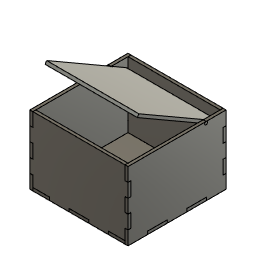
ex7 (Autodesk Fusion 360 design; units mm, degrees)
Autodesk Fusion 360 part; units mm, degrees
sketch "Sketch1" plane through (0, 0, 0) normal (1, 0, 0) x (0, 0, -1) in component "Component"
  line L0 (0, 0) -> (-100, 0)
  line L1 (-100, 0) -> (-100, 70)
  line L2 (-100, 70) -> (0, 70)
  line L3 (0, 70) -> (0, 0)
  line L4 (0, 3) -> (-100, 3)
  line L5 (-3, -14) -> (-3, 70)
  line L6 (-97, 70) -> (-97, 0)
  line L7 (-20, 3) -> (-40, 3)
  line L8 (-40, 3) -> (-40, 0)
  line L9 (-40, 0) -> (-20, 0)
  line L10 (-20, 0) -> (-20, 3)
  line L11 (-60, 3) -> (-80, 3)
  line L12 (-80, 3) -> (-80, 0)
  line L13 (-80, 0) -> (-60, 0)
  line L14 (-60, 0) -> (-60, 3)
  line L15 (-97, 14) -> (-100, 14)
  line L16 (-100, 14) -> (-100, 28)
  line L17 (-100, 28) -> (-97, 28)
  line L18 (-97, 28) -> (-97, 14)
  line L19 (-100, 42) -> (-97, 42)
  line L20 (-97, 42) -> (-97, 56)
  line L21 (-97, 56) -> (-100, 56)
  line L22 (-100, 56) -> (-100, 42)
  line L23 (0, 56) -> (-3, 56)
  line L24 (-3, 56) -> (-3, 42)
  line L25 (-3, 42) -> (0, 42)
  line L26 (0, 42) -> (0, 56)
  line L27 (-3, 28) -> (0, 28)
  line L28 (0, 28) -> (0, 14)
  line L29 (0, 14) -> (-3, 14)
  line L30 (-3, 14) -> (-3, 28)
  circle A0 centre (-20.404, 68.5087) radius 1.5
  dimension "d5" = 100
  dimension "d6" = 70
  dimension "d9" = 3
  dimension "d10" = 3
  dimension "d11" = 3
  dimension "d12" = 14
  dimension "d13" = 14
  dimension "d14" = 14
  dimension "d15" = 14
  dimension "d16" = 14
  dimension "d17" = 14
  dimension "d18" = 14
  dimension "d19" = 14
  dimension "d20" = 20
  dimension "d21" = 20
  dimension "d22" = 20
  dimension "d23" = 20
  dimension "d67" = 3
  constraint horizontal L0
  constraint vertical L1
  constraint horizontal L2
  constraint vertical L3
  constraint coincident L0.start L3.end
  constraint coincident L1 L4.end
  constraint perpendicular L1 L4
  constraint coincident L2 L5.end
  constraint perpendicular L2 L5
  constraint coincident L2 L6.start
  constraint coincident L0 L6.end
  constraint perpendicular L0 L6
  constraint horizontal L7
  constraint vertical L8
  constraint horizontal L9
  constraint vertical L10
  constraint coincident L0 L8.end
  constraint coincident L4 L7.start
  constraint horizontal L11
  constraint vertical L12
  constraint horizontal L13
  constraint vertical L14
  constraint coincident L0 L12.end
  constraint coincident L4 L11.start
  constraint horizontal L15
  constraint vertical L16
  constraint horizontal L17
  constraint vertical L18
  constraint coincident L1 L16.end
  constraint coincident L6 L15.start
  constraint horizontal L19
  constraint vertical L20
  constraint horizontal L21
  constraint vertical L22
  constraint coincident L6 L20.end
  constraint coincident L1 L19.start
  constraint horizontal L23
  constraint vertical L24
  constraint horizontal L25
  constraint vertical L26
  constraint coincident L5 L24.end
  constraint coincident L3 L23.start
  constraint horizontal L27
  constraint vertical L28
  constraint horizontal L29
  constraint vertical L30
  constraint coincident L3 L28.end
  constraint midpoint L5 L27.start
  measures "d5" distance of L0.start L0.end
  measures "d6" distance of L0.end L1.end
  measures "d9" distance of L0 L4
  measures "d10" distance of L3 L5
  measures "d11" distance of L1 L6
  measures "d12" distance of L0 L29
  measures "d13" distance of L27 L29
  measures "d14" distance of L25 L27
  measures "d15" distance of L23 L25
  measures "d16" distance of L19 L21
  measures "d17" distance of L17 L19
  measures "d18" distance of L16.end L15
  measures "d19" distance of L0 L15
  measures "d20" distance of L3 L10
  measures "d21" distance of L8 L10
  measures "d22" distance of L8 L14
  measures "d23" distance of L12 L14
  measures "d67" diameter of A0
extrude "Extrude1" add sketch "Sketch1" against normal blind 3 contours L0 L4 L5 L10 | L0 L4 L8 L14 | L0 L3 L4 L5 | L2 L4 L5 L6 L7 L11 L18 L20 L24 L30 A0 | L3 L4 L5 L29 | L0 L4 L6 L12 | L0 L1 L4 L6 | L3 L5 L25 L27 | L1 L4 L6 L15 | L2 L3 L5 L23 | L1 L6 L17 L19 | L2 A0 | L1 L2 L6 L21 picked at (-20.3416, 67.7795) makes body 1 in component "Component"
sketch "Sketch1 (2)" plane through (0, 0, 0) normal (0, 0, 1) x (1, 0, 0) in component "Component'"
  line L0 (-3, 0) -> (97, 0)
  line L1 (97, 0) -> (97, 70)
  line L2 (97, 70) -> (-3, 70)
  line L3 (-3, 70) -> (-3, 0)
  line L4 (0, 70) -> (0, 0)
  line L5 (94, 70) -> (94, 0)
  line L6 (97, 3) -> (-3, 3)
  line L7 (-3, 14) -> (0, 14)
  line L8 (0, 14) -> (0, 28)
  line L9 (0, 28) -> (-3, 28)
  line L10 (-3, 28) -> (-3, 14)
  line L11 (0, 42) -> (-3, 42)
  line L12 (-3, 42) -> (-3, 56)
  line L13 (-3, 56) -> (0, 56)
  line L14 (0, 56) -> (0, 42)
  line L15 (17, 3) -> (37, 3)
  line L16 (37, 3) -> (37, 0)
  line L17 (37, 0) -> (17, 0)
  line L18 (17, 0) -> (17, 3)
  line L19 (57, 3) -> (77, 3)
  line L20 (77, 3) -> (77, 0)
  line L21 (77, 0) -> (57, 0)
  line L22 (57, 0) -> (57, 3)
  line L23 (94, 14) -> (97, 14)
  line L24 (97, 14) -> (97, 28)
  line L25 (97, 28) -> (94, 28)
  line L26 (94, 28) -> (94, 14)
  line L27 (97, 42) -> (94, 42)
  line L28 (94, 42) -> (94, 56)
  line L29 (94, 56) -> (97, 56)
  line L30 (97, 56) -> (97, 42)
  dimension "d26" = 100
  dimension "d27" = 70
  dimension "d28" = 3
  dimension "d29" = 3
  dimension "d30" = 3
  dimension "d31" = 14
  dimension "d32" = 14
  dimension "d33" = 14
  dimension "d34" = 14
  dimension "d35" = 14
  dimension "d36" = 14
  dimension "d37" = 14
  dimension "d38" = 14
  dimension "d39" = 20
  dimension "d40" = 20
  dimension "d41" = 20
  dimension "d42" = 20
  constraint horizontal L0
  constraint vertical L1
  constraint horizontal L2
  constraint vertical L3
  constraint coincident L2 L4.start
  constraint coincident L0 L4.end
  constraint perpendicular L0 L4
  constraint coincident L2 L5.start
  constraint coincident L0 L5.end
  constraint coincident L1 L6.start
  constraint coincident L3 L6.end
  constraint vertical L5
  constraint horizontal L6
  constraint horizontal L7
  constraint vertical L8
  constraint horizontal L9
  constraint vertical L10
  constraint coincident L4 L8.end
  constraint coincident L3 L7.start
  constraint horizontal L11
  constraint vertical L12
  constraint horizontal L13
  constraint vertical L14
  constraint coincident L3 L12.end
  constraint coincident L4 L11.start
  constraint horizontal L15
  constraint vertical L16
  constraint horizontal L17
  constraint vertical L18
  constraint coincident L0 L16.end
  constraint coincident L6 L15.start
  constraint horizontal L19
  constraint vertical L20
  constraint horizontal L21
  constraint vertical L22
  constraint coincident L0 L20.end
  constraint coincident L6 L19.start
  constraint horizontal L23
  constraint vertical L24
  constraint horizontal L25
  constraint vertical L26
  constraint coincident L1 L24.end
  constraint coincident L5 L23.start
  constraint horizontal L27
  constraint vertical L28
  constraint horizontal L29
  constraint vertical L30
  constraint coincident L5 L28.end
  constraint coincident L1 L27.start
  measures "d26" distance of L0.start L0.end
  measures "d27" distance of L0.start L2.end
  measures "d28" distance of L3 L4
  measures "d29" distance of L1 L5
  measures "d30" distance of L0 L6
  measures "d31" distance of L0 L7
  measures "d32" distance of L7 L9
  measures "d33" distance of L9 L11
  measures "d34" distance of L11 L13
  measures "d35" distance of L27 L29
  measures "d36" distance of L25 L27
  measures "d37" distance of L23 L25
  measures "d38" distance of L0 L23
  measures "d39" distance of L3 L18
  measures "d40" distance of L16 L18
  measures "d41" distance of L16 L22
  measures "d42" distance of L20 L22
extrude "Extrude1'" add sketch "Sketch1 (2)" along normal blind 3 separate body contours L0 L6 L15 L16 L17 L18 | L2 L4 L5 L6 L8 L14 L15 L19 L26 L28 | L3 L4 L7 L8 L9 L10 | L0 L6 L19 L20 L21 L22 | L3 L4 L11 L12 L13 L14 | L1 L5 L23 L24 L25 L26 | L1 L5 L27 L28 L29 L30 makes body 2 in component "Component'"
copy_body "CopyPasteBodies1" bodies 2 makes body 3 in component "Component"
move_body "Move1" bodies 3 to x (1, 0, 0) y (0, 1, 0) z (0, 0, 1) at (0, 0, 97) in component "Component"
copy_body "CopyPasteBodies2" bodies 1 makes body 4 in component "Component"
move_body "Move2" bodies 4 to x (1, 0, 0) y (0, 1, 0) z (0, 0, 1) at (97, 0, 0) in component "Component"
sketch "Sketch1 (3)" plane through (0, 0, 0) normal (0, 1, 0) x (1, 0, 0) in component "Component''"
  line L0 (-3, 0) -> (97, 0)
  line L1 (97, 0) -> (97, -100)
  line L2 (97, -100) -> (-3, -100)
  line L3 (-3, -100) -> (-3, 0)
  line L4 (-3, -3) -> (97, -3)
  line L5 (94, 0) -> (94, -100)
  line L6 (-3, -97) -> (97, -97)
  line L7 (0, 0) -> (0, -100)
  line L8 (17, -97) -> (37, -97)
  line L9 (37, -97) -> (37, -100)
  line L10 (37, -100) -> (17, -100)
  line L11 (17, -100) -> (17, -97)
  line L12 (57, -97) -> (77, -97)
  line L13 (77, -97) -> (77, -100)
  line L14 (77, -100) -> (57, -100)
  line L15 (57, -100) -> (57, -97)
  line L16 (0, -80) -> (-3, -80)
  line L17 (-3, -80) -> (-3, -60)
  line L18 (-3, -60) -> (0, -60)
  line L19 (0, -60) -> (0, -80)
  line L20 (0, -40) -> (-3, -40)
  line L21 (-3, -40) -> (-3, -20)
  line L22 (-3, -20) -> (0, -20)
  line L23 (0, -20) -> (0, -40)
  line L24 (94, -20) -> (97, -20)
  line L25 (97, -20) -> (97, -40)
  line L26 (97, -40) -> (94, -40)
  line L27 (94, -40) -> (94, -20)
  line L28 (94, -60) -> (97, -60)
  line L29 (97, -60) -> (97, -80)
  line L30 (97, -80) -> (94, -80)
  line L31 (94, -80) -> (94, -60)
  line L32 (17, 0) -> (37, 0)
  line L33 (37, 0) -> (37, -3)
  line L34 (37, -3) -> (17, -3)
  line L35 (17, -3) -> (17, 0)
  line L36 (57, 0) -> (77, 0)
  line L37 (77, 0) -> (77, -3)
  line L38 (77, -3) -> (57, -3)
  line L39 (57, -3) -> (57, 0)
  dimension "d45" = 3
  dimension "d46" = 3
  dimension "d47" = 3
  dimension "d48" = 3
  dimension "d49" = 20
  dimension "d50" = 20
  dimension "d51" = 20
  dimension "d52" = 20
  dimension "d53" = 20
  dimension "d54" = 20
  dimension "d55" = 20
  dimension "d56" = 20
  dimension "d57" = 20
  dimension "d58" = 20
  dimension "d59" = 20
  dimension "d60" = 20
  dimension "d61" = 20
  dimension "d62" = 20
  dimension "d63" = 20
  dimension "d64" = 20
  constraint horizontal L0
  constraint vertical L1
  constraint horizontal L2
  constraint vertical L3
  constraint coincident L3 L4.start
  constraint coincident L1 L4.end
  constraint perpendicular L1 L4
  constraint coincident L0 L5.start
  constraint coincident L2 L5.end
  constraint perpendicular L2 L5
  constraint coincident L3 L6.start
  constraint coincident L1 L6.end
  constraint perpendicular L1 L6
  constraint coincident L0 L7.start
  constraint coincident L2 L7.end
  constraint perpendicular L2 L7
  constraint horizontal L8
  constraint vertical L9
  constraint horizontal L10
  constraint vertical L11
  constraint coincident L2 L9.end
  constraint coincident L6 L8.start
  constraint horizontal L12
  constraint vertical L13
  constraint horizontal L14
  constraint vertical L15
  constraint coincident L2 L13.end
  constraint coincident L6 L12.start
  constraint horizontal L16
  constraint vertical L17
  constraint horizontal L18
  constraint vertical L19
  constraint coincident L3 L17.end
  constraint coincident L7 L16.start
  constraint horizontal L20
  constraint vertical L21
  constraint horizontal L22
  constraint vertical L23
  constraint coincident L3 L21.end
  constraint coincident L7 L20.start
  constraint horizontal L24
  constraint vertical L25
  constraint horizontal L26
  constraint vertical L27
  constraint coincident L1 L25.end
  constraint coincident L5 L24.start
  constraint horizontal L28
  constraint vertical L29
  constraint horizontal L30
  constraint vertical L31
  constraint coincident L1 L29.end
  constraint coincident L5 L28.start
  constraint horizontal L32
  constraint vertical L33
  constraint horizontal L34
  constraint vertical L35
  constraint coincident L4 L33.end
  constraint coincident L0 L32.start
  constraint horizontal L36
  constraint vertical L37
  constraint horizontal L38
  constraint vertical L39
  constraint coincident L4 L37.end
  constraint coincident L0 L36.start
  measures "d45" distance of L0 L4
  measures "d46" distance of L1 L5
  measures "d47" distance of L2 L6
  measures "d48" distance of L3 L7
  measures "d49" distance of L3 L11
  measures "d50" distance of L9 L11
  measures "d51" distance of L9 L15
  measures "d52" distance of L13 L15
  measures "d53" distance of L2 L16
  measures "d54" distance of L16 L18
  measures "d55" distance of L18 L20
  measures "d56" distance of L20 L22
  measures "d57" distance of L24 L26
  measures "d58" distance of L26 L28
  measures "d59" distance of L28 L30
  measures "d60" distance of L2 L30
  measures "d61" distance of L3 L35
  measures "d62" distance of L33 L35
  measures "d63" distance of L33 L39
  measures "d64" distance of L37 L39
extrude "Extrude1''" add sketch "Sketch1 (3)" along normal blind 3 separate body contours L0 L4 L7 L35 | L4 L5 L6 L7 L8 L12 L19 L23 L27 L31 L34 L38 | L3 L7 L20 L21 L22 L23 | L0 L4 L33 L39 | L3 L7 L16 L17 L18 L19 | L0 L4 L5 L37 | L2 L6 L7 L11 | L1 L5 L24 L25 L26 L27 | L2 L6 L9 L15 | L1 L5 L28 L29 L30 L31 | L2 L5 L6 L13 makes body 5 in component "Component''"
extrude "Extrude2" cut sketch "Sketch1" along normal blind 112 and the other way blind 5 contours L2 A0 picked at (-20.3416, 67.7795) bodies 1 4 in component "Component"
sketch "Sketch1 (4)" plane through (0, 70, 0) normal (0, 1, 0) x (-1, 0, 0) in component "Component'''"
  line L0 (0, 20.5654) -> (3, 20.5654)
  line L1 (3, 20.5654) -> (3, 100)
  line L2 (3, 100) -> (0, 100)
  line L3 (0, 100) -> (0, 20.5654)
  line L4 (0, 3) -> (-94, 3)
  line L5 (-94, 3) -> (-94, 97)
  line L6 (-94, 97) -> (0, 97)
  line L7 (0, 97) -> (0, 3)
  line L8 (-94, 3) -> (-94, 20.4)
  circle A0 through (-94, 21.9, -1.5) (-94, 19.65, -0.201) (-94, 19.65, -2.799)
  line L9 (0, 3) -> (0, 20.4)
  circle A1 through (0, 21.9, -1.5) (0, 19.65, -0.201) (0, 19.65, -2.799)
  point P0 (0, 3)
  dimension "d74" = 17.4
  dimension "d76" = 3
  dimension "d95" = 17.4
  dimension "d96" = 3
  constraint horizontal L4
  constraint vertical L5
  constraint horizontal L6
  constraint vertical L7
  constraint coincident P0 L4.start
  constraint perpendicular L4 L8
  constraint perpendicular L4 L9
  measures "d74" distance of L4.end L8.end
  measures "d95" distance of P0 L9.end
extrude "Extrude1'''" add sketch "Sketch1 (4)" against normal blind 3 separate body contours L3 L4 L5 L6 L7 L8 L9 makes body 6 in component "Component'''"
sketch "Sketch2" plane through (94, 0, 0) normal (1, 0, 0) x (0, 0, -1) in component "Component"
  line L0 (-3, 70) -> (-97, 70)
  line L1 (-97, 70) -> (-97, 67)
  line L2 (-97, 67) -> (-3, 67)
  line L3 (-3, 67) -> (-3, 70)
  circle A0 centre (-20.4, 68.5) radius 1.5
  constraint tangent L0 A0
sketch "Sketch3" plane through (0, 70, 0) normal (0, 1, 0) x (-1, 0, 0) in component "Component"
  line L0 (0, 97) -> (-94, 97)
  line L1 (-94, 97) -> (-94, 3)
  line L2 (-94, 3) -> (0, 3)
  line L3 (0, 3) -> (0, 97)
sketch "Sketch4" plane through (0, 70, 0) normal (0, 1, 0) x (-1, 0, 0) in component "Component"
sketch "Sketch5" plane through (0, 70, 0) normal (0, 1, 0) x (-1, 0, 0) in component "Component"
  circle A0 through (-94, 21.9, -1.5) (-94, 19.65, -0.201) (-94, 19.65, -2.799)
  point P0 (-94, 20.4)
sketch "Sketch6" plane through (94, 68.5, 20.4) normal (-1, 0, 0) x (0, -1, 0) in component "Component"
extrude "Extrude1''''" add sketch "Sketch1 (4)" along normal blind -3 and the other way blind -97 separate body contours A0 in plane through (94, 70, 0) normal (-1, 0, 0) makes body 7 in component "Component''''"
extrude "Extrude2'" cut sketch "Sketch1 (4)" along normal blind 94 contours A0 in plane through (94, 70, 0) normal (-1, 0, 0) bodies 7 makes body 8 at (95, 67.987, 18.9905) in component "Component''''"
move_body "Move1'" bodies 6 to x (1, 0, 0) y (0, 0.866025, -0.5) z (0, 0.5, 0.866025) at (0, -1.0227, 36.9831) in component "Component'''"
sketch "Sketch1 (5)" plane through (0, 0, 0) normal (1, 0, 0) x (0, 0, -1)
component "Component" placed x (1, 0, 0) y (0, 1, 0) z (0, 0, 1) at (0, 0, 0)
component "Component'" placed x (1, 0, 0) y (0, 1, 0) z (0, 0, 1) at (0, 0, 0) in component "Component"
component "Component''" placed x (1, 0, 0) y (0, 1, 0) z (0, 0, 1) at (0, 0, 0) in component "Component"
component "Component'''" placed x (1, 0, 0) y (0, 1, 0) z (0, 0, 1) at (0, 0, 0) in component "Component"
component "Component''''" placed x (1, 0, 0) y (0, 1, 0) z (0, 0, 1) at (0, 0, 0) in component "Component"
equation "len = 100 mm"
equation "base = 100 mm"
equation "h = 70 mm"
equation "d5 = len"
equation "d6 = h"
equation "thic = 3 mm"
equation "nt = 2"
equation "d9 = thic"
equation "d10 = thic"
equation "d11 = thic"
equation "d12 = h / ( 2 * nt + 1 )"
equation "d13 = d12"
equation "d14 = d12"
equation "d15 = d12"
equation "d16 = d15"
equation "d17 = d14"
equation "d18 = d13"
equation "d19 = d12"
equation "d20 = len / ( 2 * nt + 1 )"
equation "d21 = d20"
equation "d22 = d20"
equation "d23 = d20"
equation "d26 = len"
equation "d27 = h"
equation "d28 = thic"
equation "d29 = thic"
equation "d30 = thic"
equation "d31 = h / ( 2 * nt + 1 )"
equation "d32 = d31"
equation "d33 = d31"
equation "d34 = d31"
equation "d35 = d34"
equation "d36 = d33"
equation "d37 = d32"
equation "d38 = d31"
equation "d39 = len / ( 2 * nt + 1 )"
equation "d40 = d39"
equation "d41 = d39"
equation "d42 = d39"
equation "d45 = thic"
equation "d46 = thic"
equation "d47 = thic"
equation "d48 = thic"
equation "d49 = len / ( 2 * nt + 1 )"
equation "d50 = d49"
equation "d51 = d50"
equation "d52 = d49"
equation "d53 = base / ( 2 * nt + 1 )"
equation "d54 = d53"
equation "d55 = d53"
equation "d56 = d53"
equation "d57 = d56"
equation "d58 = d55"
equation "d59 = d54"
equation "d60 = d53"
equation "d61 = d49"
equation "d62 = d50"
equation "d63 = d51"
equation "d64 = d52"
